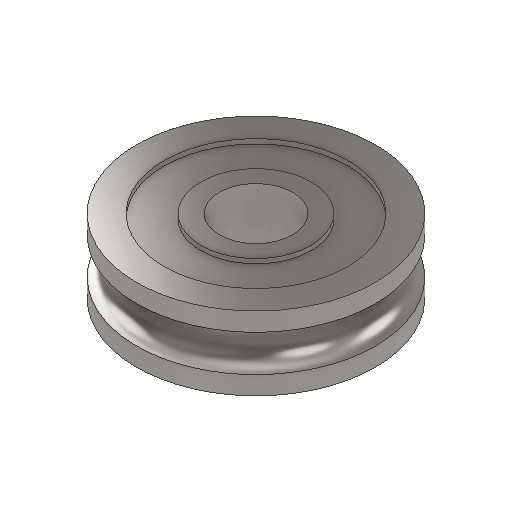
# Autodesk Inventor part: BearingU604
Saved by Autodesk Inventor 2026.2 (Build 302298000, 298)
## iProperties
Created: 2026-03-28
Part Number: BearingU604
Material: Steel, Alloy
Document SubType Name: Modeling
Designer: gaoet
Density: 7.73 g/cm^3
Appearance: Semi-Polished
Author: gaoet
Autodesk Inventor part; units mm, degrees
ref_plane "YZ Plane" through (0, 0, 0) normal (1, 0, 0) x (0, 1, 0)
ref_plane "XZ Plane" through (0, 0, 0) normal (0, 1, 0) x (-1, 0, 0)
ref_plane "XY Plane" through (0, 0, 0) normal (0, 0, 1) x (1, 0, 0)
sketch "Sketch1" plane through (0, 0, 0) normal (0, 0, 1) x (1, 0, 0)
  line L0 (0, 0) -> (0, 5.0023) construction
  line L1 (2, 0) -> (6.5, 0)
  line L2 (6.5, 0) -> (6.5, 4)
  line L3 (6.5, 4) -> (2, 4)
  line L4 (2, 4) -> (2, 0)
  circle A0 centre (6.5, 2) radius 1
  line L5 (3, 4) -> (3, 3.75)
  line L6 (3, 3.75) -> (5, 3.75)
  line L7 (5, 3.75) -> (5, 4)
  line L8 (3, 0) -> (3, 0.25)
  line L9 (3, 0.25) -> (5, 0.25)
  line L10 (5, 0.25) -> (5, 0)
  point P0 (0, 2.5011)
  point P1 (6.5, 1)
  point P2 (6.5, 3)
  point P3 (3, 3.875)
  dimension "d0" = 2
  dimension "d1" = 2
  dimension "d2" = 6.5
  dimension "d3" = 4
  dimension "d5" = 0.25
  dimension "d6" = 1
  dimension "d7" = 2
  constraints: 22 end point, 6 point on line, 4 perpendicular, 3 midpoint, 3 vertical, 2 equal length, 2 parallel, 1 centre point, 1 horizontal, 1 horizontal alignment
  measures "d0" diameter of A0
  measures "d1" distance from line of point (0, 2.501) L4
  measures "d2" distance between parallel lines of L0 L2
  measures "d3" distance of L3.end L1.start
  measures "d5" distance of L5.end L5.start
  measures "d6" distance from line of L4 point (3, 3.875)
  measures "d7" distance of L5.end L6.end
revolve "Revolution1" add sketch "Sketch1" angle 360 about axis through (0, 0, 0) along (0, 1, 0) contours L4 L3 L5 L6 L7 L2 A0 L1 L10 L9 L8
body "Solid1"
